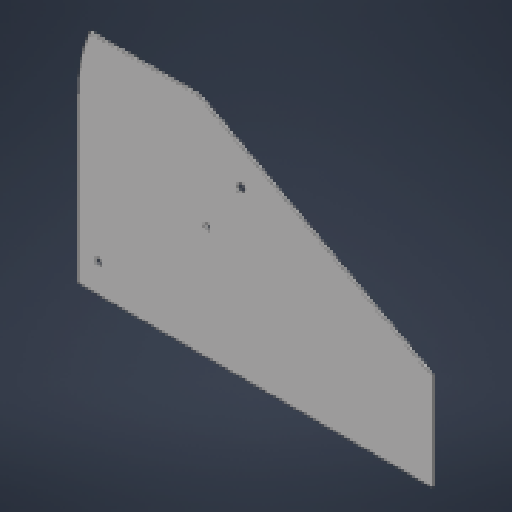
# Autodesk Inventor part: стенка
Saved by Autodesk Inventor 2025 (Build 290162000, 162)
## iProperties
Created: 2025-10-03
Part Number: стенка
Material: Типовые
Document SubType Name: Modeling
Designer: Phantom
Density: 1 g/cm^3
Appearance: По умолчанию
Author: Phantom
Autodesk Inventor part; units mm, degrees
ref_plane "YZ Plane" through (0, 0, 0) normal (1, 0, 0) x (0, 1, 0)
ref_plane "XZ Plane" through (0, 0, 0) normal (0, 1, 0) x (-1, 0, 0)
ref_plane "XY Plane" through (0, 0, 0) normal (0, 0, 1) x (1, 0, 0)
sketch "Эскиз1" plane through (0, 0, 0) normal (0, 0, 1) x (1, 0, 0)
  line L0 (0, 0) -> (380, 0)
  line L1 (380, 0) -> (380, 227)
  line L2 (380, 227) -> (0, 227)
  line L3 (0, 227) -> (0, 0)
  dimension "d0" = 380
  dimension "d1" = 227
  constraints: 8 end point, 2 parallel, 1 horizontal, 1 perpendicular
  measures "d0" distance of L2.end L1.end
  measures "d1" distance of L1.end L0.end
extrude "Выдавливание1" add sketch "Эскиз1" along normal blind 2
sketch "Эскиз2" plane through (0, 0, 2) normal (0, 0, 1) x (1, 0, 0)
  arc A0 (28.7106, 220.3235) -> (184.1593, 0) centre (184.1593, 165) ccw projected
  line L0 (380, 0) -> (380, 227) projected
  line L1 (380, 227) -> (0, 227) projected
  line L2 (0, 227) -> (0, 0) projected
  line L3 (0, 0) -> (380, 0) projected
  line L4 (19.1593, 227.9564) -> (19.1593, -26.9054)
  line L5 (0, 227) -> (0, 0) projected
  circle A1 centre (184.1593, 165) radius 165
  point P0 (19.1593, 165)
  point P1 (24, 227)
  point P2 (19.1593, 0)
  point P3 (19.1593, 227)
  point P4 (184.1593, 0)
  point P5 (28.7106, 220.3235)
  point P6 (31.2508, 227)
  constraints: 2 end point, 1 centre point, 1 coincident, 1 concentric, 1 parallel, 1 tangent
extrude "Выдавливание2" cut sketch "Эскиз2" against normal blind 10 contours A0 L4 L1 A1 | L4 L3 L2 L1
sketch "Эскиз3" plane through (0, 0, 0) normal (0, 0, -1) x (-1, 0, 0)
  line L0 (-232.105, -3.3128) -> (-396.3335, -92) projected
  line L1 (-142.3437, 227) -> (-503.0133, 32.2299)
  line L2 (-14.4537, 180) -> (-380, 180) projected
  line L3 (-14.4537, 180) -> (-380, 180) projected
  line L4 (-380, 0) -> (-380, 180) projected
  line L5 (-14.1593, 0) -> (-380, 0) projected
  line L6 (-14.1593, 0) -> (-14.1593, 170) projected
  arc A0 (-14.1593, 170) -> (-14.4537, 180) centre (-184.1593, 170) ccw projected
  line L7 (-19.1593, 0) -> (-19.1593, 165) projected
  arc A1 (-19.1593, 165) -> (-31.2508, 227) centre (-184.1593, 165) ccw projected
  line L8 (-380, 227) -> (-31.2508, 227) projected
  line L9 (-380, 0) -> (-380, 227) projected
  line L10 (-19.1593, 0) -> (-380, 0) projected
  point P0 (0, 0)
  point P1 (-380, 98.66)
  dimension "d6" = 160
  constraints: 2 end point, 1 parallel, 1 point on line, 1 other
  measures "d6" distance between parallel lines of L0 L1
extrude "Выдавливание3" cut sketch "Эскиз3" against normal blind 10 contours L1 L2 L9 L8 | L1 L4 L2
sketch "Эскиз4" plane through (0, 0, 0) normal (0, 0, -1) x (-1, 0, 0)
  circle A0 centre (-150.9975, 115.172) radius 3 projected
  circle A1 centre (-150.9975, 115.172) radius 3.1
  circle A2 centre (-184.1593, 165) radius 3.1 projected
  circle A3 centre (-184.1593, 165) radius 3.1
  arc A4 (-37.1443, 30.0275) -> (-37.7482, 26.6179) centre (-39.8587, 28.75) ccw projected
  circle A5 centre (-39.8587, 28.75) radius 3.5
  point P0 (0, 0)
  dimension "d9" = 6.2
  dimension "d10" = 6.2
  dimension "d11" = 7
  constraints: 3 centre point, 3 coincident
  measures "d9" diameter of A1
  measures "d10" diameter of A3
  measures "d11" diameter of A5
extrude "Выдавливание5" cut sketch "Эскиз4" against normal blind 10 contours A0 | A2 | A5
sketch "Эскиз5" plane through (0, 0, 0) normal (0, 0, -1) x (-1, 0, 0)
  circle A0 centre (-184.1593, 165) radius 3.1
  circle A1 centre (-185.6251, 167.2025) radius 3.5
  circle A2 centre (-150.9975, 115.172) radius 3 projected
  circle A3 centre (-150.9975, 115.172) radius 62.5
  circle A4 centre (-182.6583, 169.0593) radius 3.5
  line L0 (-182.6583, 169.0593) -> (-162.6583, 169.0593)
  line L1 (-182.6583, 169.0593) -> (-162.6583, 169.0593) construction
  line L2 (-162.6583, 169.0593) -> (-162.6583, 176.0593)
  line L3 (-162.6583, 176.0593) -> (-181, 176.0593)
  circle A5 centre (-165.1036, 176.0593) radius 3.5
  point P0 (0, 0)
  point P1 (-187.1037, 164.0302)
  point P2 (-182.1279, 167.3417)
  point P3 (-185.8413, 167.604)
  point P4 (-185.7497, 170.7003)
  dimension "d20" = 7
  dimension "d21" = 20
  dimension "d22" = 0
  dimension "d23" = 7
  dimension "d24" = 7
  constraints: 8 end point, 4 centre point, 3 point on circle, 2 horizontal, 2 perpendicular, 1 coincident, 1 collinear, 1 point on line, 6 other
  measures "d20" diameter of A4
  measures "d21" distance of L0.start L0.end
  measures "d22" distance between parallel lines of L0 L1
  measures "d23" distance of L0.end L2.end
  measures "d24" diameter of A5
extrude "Выдавливание6" cut sketch "Эскиз5" against normal blind 7 contours A4 A1 A0 | A0 A1 L0 A4 | A1 A3 A0 | A1 A4 A3 A0 | A0 A3 A1 | L0 A3 A4 | A3 A1 A4 A0 | A3 A4 A0 | A0 A4 A1 A3 | A1 A4 A3 | A5 L3 A3 | A3 L3 L2 A5 | L2 L3 A3 A5 | A3 L3 A5 picked at (-181.7788, 166.0755) picked at (-184.2655, 167.3284) picked at (-187.1066, 167.9908) picked at (-185.4271, 167.6129) picked at (-185.0911, 169.2148)
equation "\"d16\" = d24"
